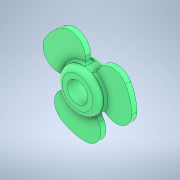
# Autodesk Inventor part: fan
Saved by Autodesk Inventor 2021 (Build 250183000, 183)
## iProperties
Created: 2021-07-30
Part Number: fan
Material: PPS Plastic
Document SubType Name: Modeling
Designer: Shammy Haider
Mass: 0.0651766 g
Surface Area: 1.50321 cm^2
Volume: 0.0398146 cm^3
Density: 1.637 g/cm^3
Appearance: Smooth - White
Author: Shammy Haider
Autodesk Inventor part; units mm, degrees
ref_plane "YZ Plane" through (0, 0, 0) normal (1, 0, 0) x (0, 1, 0)
ref_plane "XZ Plane" through (0, 0, 0) normal (0, 1, 0) x (-1, 0, 0)
ref_plane "XY Plane" through (0, 0, 0) normal (0, 0, 1) x (1, 0, 0)
sketch "Sketch1" plane through (0, 0, 0) normal (0, 0, 1) x (1, 0, 0)
  circle A0 centre (0, 0) radius 2
  circle A1 centre (0, 0) radius 1
  dimension "d0" = 4
  dimension "d1" = 2
  constraints: 2 centre point, 2 coincident
  measures "d0" diameter of A0
  measures "d1" diameter of A1
extrude "Extrusion1" add sketch "Sketch1" along normal mid plane 2
sketch "Sketch2" plane through (0, 0, 0) normal (0, 0, 1) x (1, 0, 0)
  point P0 (0, 0)
sketch "Sketch3" plane through (0, 0, 0) normal (0, 1, 0) x (-1, 0, 0)
  line L0 (2, 0.25) -> (4.5, 0.25)
  line L1 (4.5, 0.25) -> (4.5, -0.25)
  line L2 (4.5, -0.25) -> (2, -0.25)
  line L3 (2, -0.25) -> (2, 0.25)
  line L4 (2, 1) -> (-2, 1) projected
  line L5 (0, 0) -> (0, -2.5781)
  dimension "d4" = 0.5
  dimension "d5" = 2.5
  dimension "d6" = 0.75
  dimension "d15" = 4
  constraints: 10 end point, 2 parallel, 1 horizontal, 1 perpendicular, 1 vertical
  measures "d4" distance of L0.end L1.end
  measures "d5" distance of L1.end L2.end
  measures "d6" distance between parallel lines of L0 L4
  measures "d15" diameter of L3 L5
revolve "Revolution1" add sketch "Sketch3" angle 90 about axis through (0, 0, 0) along (0, 0, -1)
fillet "Fillet1" radius 1.5 2 edges at (0, 4.5, 0) (-4.5, 0, 0)
fillet "Fillet2" radius 0.2 4 edges at (-2, 0, 0) (-1.4142, 1.4142, -0.25) (-1.4142, 1.4142, 0.25) (0, 2, 0)
pattern_circular "Circular Pattern1" count 3 over 360 about axis through (0, 0, 0) along (0, 0, 1) of "Revolution1", "Fillet1", "Fillet2"
fillet "Fillet3" radius 0.5 1 edges at (-2, 0, 1)
fillet "Fillet3" radius 0.5 1 edges at (-2, 0, -1)
equation "\"d1\" = 0.5 * d0"
body "Solid1"
